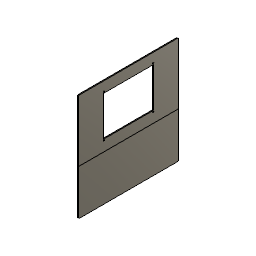
dehumidifier panel for last resort fila cab (Autodesk Fusion 360 design; units mm, degrees)
part number: 2026-08-29-23-02-58-721
Autodesk Fusion 360 part; units mm, degrees
sketch "Sketch1" plane through (0, 0, 0) normal (1, 0, 0) x (0, 1, 0)
  line L0 (142, -152) -> (-142, -152)
  line L1 (-142, -152) -> (-142, 152)
  line L2 (-142, 152) -> (142, 152)
  line L3 (142, 152) -> (142, -152)
  line L4 (142, -152) -> (-142, 152) construction
  line L5 (-142, -152) -> (142, 152) construction
  line L6 (0, 0) -> (0, 65) construction
  line L7 (71.2, 8.8) -> (-71.2, 8.8)
  line L8 (-71.2, 8.8) -> (-71.2, 121.2)
  line L9 (-71.2, 121.2) -> (71.2, 121.2)
  line L10 (71.2, 121.2) -> (71.2, 8.8)
  line L11 (71.2, 8.8) -> (-71.2, 121.2) construction
  line L12 (-71.2, 8.8) -> (71.2, 121.2) construction
  line L13 (70, 5) -> (-70, 5) construction
  line L14 (-70, 5) -> (-70, 125) construction
  line L15 (-70, 125) -> (70, 125) construction
  line L16 (70, 125) -> (70, 5) construction
  line L17 (70, 5) -> (-70, 125) construction
  line L18 (-70, 5) -> (70, 125) construction
  line L19 (0, 152) -> (0, 142) construction
  circle A0 centre (-70, 125) radius 1.7
  circle A1 centre (70, 125) radius 1.7
  circle A2 centre (70, 5) radius 1.7
  circle A3 centre (-70, 5) radius 1.7
  point P0 (0, 65)
  point P1 (0, 65)
  dimension "d1" = 304
  dimension "d2" = 284
  dimension "d3" = 65
  dimension "d4" = 142.4
  dimension "d5" = 112.4
  dimension "d6" = 140
  dimension "d7" = 120
  dimension "d8" = 10
  dimension "d9" = 3.4
  dimension "d10" = 3.4
  dimension "d11" = 3.4
  dimension "d12" = 3.4
  constraint horizontal L0
  constraint perpendicular L0 L1
  constraint parallel L0 L2
  constraint parallel L1 L3
  constraint coincident L4 L6.start
  constraint coincident L5 L6.start
  constraint coincident L6.start origin
  constraint vertical L6
  constraint horizontal L7
  constraint perpendicular L7 L8
  constraint parallel L7 L9
  constraint parallel L8 L10
  constraint coincident L11 P1
  constraint coincident L12 P1
  constraint coincident P1 P0
  constraint horizontal L13
  constraint perpendicular L13 L14
  constraint parallel L13 L15
  constraint parallel L14 L16
  constraint coincident L17 P1
  constraint coincident L18 P1
  constraint midpoint L2 L19.start
  constraint perpendicular L2 L19
  constraint coincident L14.end L15.start
  constraint coincident L15.end L16.start
  constraint coincident L13.start L16.end
  constraint coincident L13.end L14.start
  measures "d1" distance of L0.end L1.end
  measures "d2" distance of L1.end L2.end
  measures "d3" distance of L6.start P1
  measures "d4" distance of L8.end L9.end
  measures "d5" distance of L7.end L8.end
  measures "d6" distance of L14.end L15.end
  measures "d7" distance of L13.end L14.end
  measures "d8" distance of L19.start L19.end
  measures "d9" diameter of A0
  measures "d10" diameter of A1
  measures "d11" diameter of A2
  measures "d12" diameter of A3
extrude "Extrude1" add sketch "Sketch1" along normal blind 3 makes body 1
fillet "Fillet1" radius 2 4 edges at (1.5, 142, -152) (1.5, -142, -152) (1.5, -142, 152) (1.5, 142, 152) on bodies 1
fillet "Fillet1" radius 1 4 edges at (1.5, 71.2, 121.2) (1.5, 71.2, 8.8) (1.5, -71.2, 8.8) (1.5, -71.2, 121.2) on bodies 1
ref_plane "WorkPlane1" through (1.5, 0, -23) normal (0, 0, 1) x (0, -1, 0)
split "Split1" by plane through (1.5, 0, -23) normal (0, 0, 1) bodies 1 makes body 2 at (0, 118.4, 45.6)
